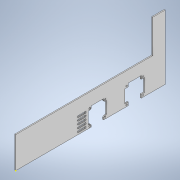
# Autodesk Inventor part: 220228 Left Side with brace
Saved by Autodesk Inventor 2022 (Build 260153000, 153)
## iProperties
Created: 2022-02-07
Part Number: 220228 Left Side with brace
Material: Generic
Document SubType Name: Modeling
Designer: josephinew
Density: 1 g/cm^3
Appearance: Default
Author: josephinew
Autodesk Inventor part; units mm, degrees
ref_plane "YZ Plane" through (0, 0, 0) normal (1, 0, 0) x (0, 1, 0)
ref_plane "XZ Plane" through (0, 0, 0) normal (0, 1, 0) x (-1, 0, 0)
ref_plane "XY Plane" through (0, 0, 0) normal (0, 0, 1) x (1, 0, 0)
sketch "Sketch1" plane through (0, 0, 0) normal (1, 0, 0) x (0, 1, 0)
  line L0 (0, 0) -> (95.25, 0)
  line L1 (95.25, 0) -> (95.25, -419.1)
  line L2 (95.25, -457.2) -> (0, -457.2)
  line L3 (0, -457.2) -> (0, 0)
  line L4 (0, -457.2) -> (196.85, -457.2)
  line L5 (196.85, -457.2) -> (196.85, -419.1)
  line L6 (196.85, -419.1) -> (95.25, -419.1)
  line L7 (0, -419.1) -> (0, -457.2)
  constraints: 16 end point, 4 parallel, 2 horizontal, 2 perpendicular
extrude "Extrusion1" add sketch "Sketch1" along normal blind 3.175
sketch "Sketch2" plane through (0, 0, 0) normal (-1, 0, 0) x (0, 0, 1)
  line L0 (-393.7, 49.9364) -> (-393.7, 10.0076)
  line L1 (-333.756, 10.0076) -> (-333.756, 49.9364)
  line L2 (-343.7636, 59.944) -> (-383.6924, 59.944)
  circle A0 centre (-388.6962, 54.9402) radius 2.159
  circle A1 centre (-338.7598, 54.9402) radius 2.159
  circle A2 centre (-388.6962, 5.0038) radius 2.159
  circle A3 centre (-338.7598, 5.0038) radius 2.159
  line L3 (-383.6924, 59.944) -> (-383.6924, 49.9364)
  line L4 (-383.6924, 49.9364) -> (-393.7, 49.9364)
  line L5 (-343.7636, 59.944) -> (-343.7636, 49.9364)
  line L6 (-343.7636, 49.9364) -> (-333.756, 49.9364)
  line L7 (-383.6924, 0) -> (-383.6924, 10.0076)
  line L8 (-383.6924, 10.0076) -> (-393.7, 10.0076)
  line L9 (-343.7636, 0) -> (-343.7636, 10.0076)
  line L10 (-343.7636, 10.0076) -> (-333.756, 10.0076)
  circle A4 centre (-273.2786, 51.7724) radius 2.54
  circle A5 centre (-273.2786, 4.63) radius 2.54
  circle A6 centre (-226.1362, 51.7724) radius 2.54
  circle A7 centre (-226.1362, 4.63) radius 2.54
  line L11 (-190.9572, 5.646) -> (-212.4456, 5.646)
  line L12 (-212.4456, 10.726) -> (-190.9572, 10.726)
  arc A8 (-190.9572, 5.646) -> (-190.9572, 10.726) centre (-190.9572, 8.186) ccw
  arc A9 (-212.4456, 10.726) -> (-212.4456, 5.646) centre (-212.4456, 8.186) ccw
  line L13 (-190.9572, 15.6282) -> (-212.4456, 15.6282)
  line L14 (-212.4456, 20.7082) -> (-190.9572, 20.7082)
  arc A10 (-190.9572, 15.6282) -> (-190.9572, 20.7082) centre (-190.9572, 18.1682) ccw
  arc A11 (-212.4456, 20.7082) -> (-212.4456, 15.6282) centre (-212.4456, 18.1682) ccw
  line L15 (-190.9572, 25.6104) -> (-212.4456, 25.6104)
  line L16 (-212.4456, 30.6904) -> (-190.9572, 30.6904)
  arc A12 (-190.9572, 25.6104) -> (-190.9572, 30.6904) centre (-190.9572, 28.1504) ccw
  arc A13 (-212.4456, 30.6904) -> (-212.4456, 25.6104) centre (-212.4456, 28.1504) ccw
  line L17 (-190.9572, 35.5926) -> (-212.4456, 35.5926)
  line L18 (-212.4456, 40.6726) -> (-190.9572, 40.6726)
  arc A14 (-190.9572, 35.5926) -> (-190.9572, 40.6726) centre (-190.9572, 38.1326) ccw
  arc A15 (-212.4456, 40.6726) -> (-212.4456, 35.5926) centre (-212.4456, 38.1326) ccw
  line L19 (-190.9572, 45.5748) -> (-212.4456, 45.5748)
  line L20 (-212.4456, 50.6548) -> (-190.9572, 50.6548)
  arc A16 (-190.9572, 45.5748) -> (-190.9572, 50.6548) centre (-190.9572, 48.1148) ccw
  arc A17 (-212.4456, 50.6548) -> (-212.4456, 45.5748) centre (-212.4456, 48.1148) ccw
  line L21 (-457.2, 0) -> (-457.2, 196.85) projected
  line L22 (-457.2, 0) -> (-393.7, 0)
  line L23 (-383.6924, 0) -> (-343.7636, 0)
  line L24 (-419.1, 95.25) -> (0, 95.25) projected
  line L25 (-4.8028, 0) -> (-4.8028, 95.25)
  line L26 (-4.8028, 95.25) -> (-457.2, 95.25)
  line L27 (-457.2, 95.25) -> (-457.2, 0)
  line L28 (-267.3803, 56.4007) -> (-232.0345, 56.4007)
  line L29 (-221.5079, 45.8741) -> (-221.5079, 10.5283)
  line L30 (-232.0345, 0) -> (-267.3803, 0)
  line L31 (-277.9086, 10.5283) -> (-277.9086, 45.8741)
  line L32 (-273.2786, 51.7724) -> (-271.5234, 49.9364)
  line L33 (-271.5234, 49.9364) -> (-270.4878, 48.8532)
  arc A18 (-268.6503, 4.5045) -> (-273.4041, 9.2583) centre (-273.2786, 4.63) ccw
  arc A19 (-226.1362, 9.2583) -> (-230.7645, 4.63) centre (-226.1362, 4.63) ccw
  arc A20 (-230.7645, 51.7724) -> (-226.1362, 47.1441) centre (-226.1362, 51.7724) ccw
  arc A21 (-273.2786, 47.1441) -> (-268.6503, 51.7724) centre (-273.2786, 51.7724) ccw
  line L34 (-268.6503, 55.1307) -> (-268.6503, 51.7724)
  line L35 (-273.2786, 47.1441) -> (-276.6386, 47.1441)
  line L36 (-230.7645, 55.1307) -> (-230.7645, 51.7724)
  line L37 (-226.1362, 47.1441) -> (-222.7779, 47.1441)
  line L38 (-221.5079, 0) -> (-230.7645, 0)
  line L39 (-230.7645, 1.27) -> (-230.7645, 4.63)
  line L40 (-226.1362, 9.2583) -> (-222.7779, 9.2583)
  line L41 (-277.9086, 0) -> (-268.6503, 0)
  line L42 (-268.6503, 1.27) -> (-268.6503, 4.7555)
  line L43 (-273.1531, 9.2583) -> (-276.6386, 9.2583)
  arc A22 (-277.9086, 10.5283) -> (-276.6386, 9.2583) centre (-276.6386, 10.5283) ccw
  arc A23 (-267.3803, 56.4007) -> (-268.6503, 55.1307) centre (-267.3803, 55.1307) ccw
  arc A24 (-276.6386, 47.1441) -> (-277.9086, 45.8741) centre (-276.6386, 45.8741) ccw
  arc A25 (-230.7645, 55.1307) -> (-232.0345, 56.4007) centre (-232.0345, 55.1307) ccw
  arc A26 (-221.5079, 45.8741) -> (-222.7779, 47.1441) centre (-222.7779, 45.8741) ccw
  arc A27 (-222.7779, 9.2583) -> (-221.5079, 10.5283) centre (-222.7779, 10.5283) ccw
  line L44 (-277.9086, 56.4007) -> (-277.7032, 56.4007)
  line L45 (-268.6503, 4.5045) -> (-268.6503, 0)
  line L46 (0, 0) -> (-457.2, 0) projected
  line L47 (-230.7645, 4.63) -> (-230.7645, 0)
  line L48 (-268.6503, 0) -> (-230.7645, 0)
  dimension "d50" = 1.4986
  dimension "d52" = 1.27
  constraints: 92 end point, 43 point on circle, 27 centre point, 16 tangent, 13 point on line, 6 parallel, 5 horizontal, 4 coincident, 4 equal radius, 4 perpendicular, 1 collinear, 1 vertical, 4 other
  measures "d50" distance of L32.end L33.end
  measures "d52" radius of A23
extrude "Extrusion2" cut sketch "Sketch2" against normal blind 25.4 contours L4 L3 L2 L5 L6 L1 L10 L9 L23 L7 L8 L0 | L45 L42 A18 L43 A22 L31 A24 L35 A21 L34 A23 L28 A25 L36 A20 L37 A26 L29 A27 L40 A19 L39 L47 L46 L30 | A0 | A1 | A2 | A3 | A4 | A5 | A6 | A7 | L11 A9 L12 A8 | L13 A11 L14 A10 | L15 A13 L16 A12 | L17 A15 L18 A14 | L19 A17 L20 A16
sketch "Sketch6" plane through (3.175, 0, 0) normal (1, 0, 0) x (0, 0, -1)
  point P0 (0, 0)
body "Solid1"
